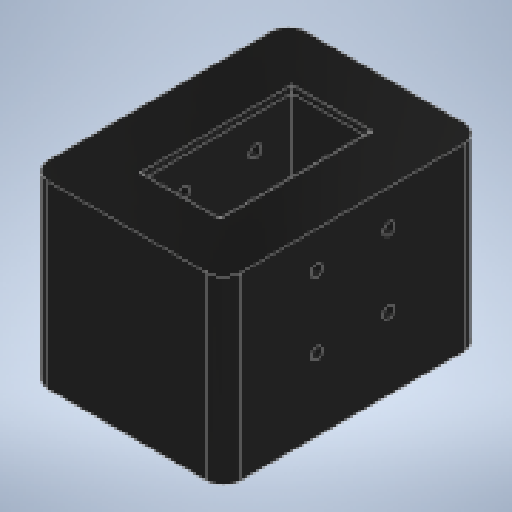
# Autodesk Inventor part: framefixpart1
Saved by Autodesk Inventor 2024 (Build 280153000, 153)
## iProperties
Created: 2025-05-28
Part Number: framefixpart1
Material: 一般
Document SubType Name: Modeling
Designer: kshau
Density: 1 g/cm^3
Appearance: 滑らか - 黒
Mass: 159.689 g
Surface Area: 260.007 cm^2
Volume: 159.689 cm^3
Author: kshau
Autodesk Inventor part; units mm, degrees
ref_plane "YZ Plane" through (0, 0, 0) normal (1, 0, 0) x (0, 1, 0)
ref_plane "XZ Plane" through (0, 0, 0) normal (0, 1, 0) x (-1, 0, 0)
ref_plane "XY Plane" through (0, 0, 0) normal (0, 0, 1) x (1, 0, 0)
sketch "スケッチ1" plane through (0, 0, 0) normal (0, 1, 0) x (-1, 0, 0)
  line L0 (0, 0) -> (53.8, 0)
  line L1 (53.8, 0) -> (53.8, -71.8)
  line L2 (53.8, -71.8) -> (0, -71.8)
  line L3 (0, -71.8) -> (0, 0)
  dimension "d0" = 53.8
  dimension "d1" = 71.8
  constraints: 8 end point, 2 parallel, 1 horizontal, 1 perpendicular
  measures "d0" distance of L0.start L0.end
  measures "d1" distance of L2.end L0.start
extrude "押し出し1" add sketch "スケッチ1" along normal blind 10
sketch "スケッチ2" plane through (0, 10, 0) normal (0, 1, 0) x (1, 0, 0)
  line L0 (-53.8, 71.8) -> (-53.8, 0) projected
  line L1 (-53.8, 0) -> (0, 0) projected
  line L2 (-26.9, 0) -> (-26.9, 71.8)
  line L3 (0, 71.8) -> (-53.8, 71.8) projected
  line L4 (-53.8, 35.9) -> (0, 35.9)
  line L5 (0, 0) -> (0, 71.8) projected
  line L6 (-26.9, 35.9) -> (-37.05, 35.9)
  line L7 (-37.05, 35.9) -> (-37.05, 56.05)
  line L8 (-37.05, 56.05) -> (-26.9, 56.05)
  line L9 (-26.9, 56.05) -> (-26.9, 35.9)
  line L10 (-37.05, 35.9) -> (-37.05, 15.75)
  line L11 (-37.05, 15.75) -> (-26.9, 15.75)
  line L12 (-16.75, 35.9) -> (-16.75, 56.05)
  line L13 (-16.75, 56.05) -> (-26.9, 56.05)
  line L14 (-16.75, 35.9) -> (-16.75, 15.75)
  line L15 (-16.75, 15.75) -> (-26.9, 15.75)
  dimension "d7" = 20.15
  dimension "d8" = 10.15
  constraints: 24 end point, 5 midpoint, 5 symmetric about line, 2 parallel, 1 horizontal, 1 perpendicular
  measures "d7" distance of L6.end L7.end
  measures "d8" distance of L7.end L8.end
extrude "押し出し2" add sketch "スケッチ2" along normal blind 40 contours L3 L2 L8 L7 L4 L0 | L4 L10 L11 L2 L1 L0 | L3 L5 L4 L12 L13 L2 | L2 L15 L14 L4 L5 L1
fillet "フィレット1" radius 5 4 edges at (0, 25, 0) (0, 25, -71.8) (-53.8, 25, -71.8) (-53.8, 25, 0)
sketch "スケッチ3" plane through (0, 0, -5) normal (1, 0, 0) x (0, 0, -1)
  line L0 (51.05, 50) -> (10.75, 50) projected
  line L1 (30.9, 50) -> (30.9, 0)
  line L2 (0, 0) -> (61.8, 0) projected
  line L3 (20.9, 50) -> (20.9, 0)
  line L4 (0, 50) -> (0, 0) projected
  line L5 (0, 10) -> (62, 10)
  line L6 (10.75, 10) -> (51.05, 10) projected
  point P0 (-5, 0)
  point P1 (20.9, 20)
  point P2 (20.9, 40)
  point P3 (40.9, 20)
  point P4 (40.9, 40)
  dimension "d12" = 10
  dimension "d13" = 10
  dimension "d14" = 10
  dimension "d15" = 20
  constraints: 6 end point, 3 point on line, 2 midpoint, 2 symmetric about line, 1 collinear, 1 vertical
  measures "d12" distance between parallel lines of L1 L3
  measures "d13" distance between parallel lines of L2 L5
  measures "d14" distance from line of L5 point (20.9, 20)
  measures "d15" distance of point (20.9, 20) point (20.9, 40)
hole "穴1" at (0, 20, -25.9) at (0, 40, -25.9) at (0, 40, -45.9) at (0, 20, -45.9) direction (-1, 0, 0) diameter 3.3 end through all
sketch "スケッチ4" plane through (0, 0, 0) normal (0, -1, 0) x (1, 0, 0)
  line L0 (-5, -71.8) -> (-48.8, -71.8) projected
  line L1 (-26.9, -71.8) -> (-26.9, 0)
  line L2 (-48.8, 0) -> (-5, 0) projected
  line L3 (-53.8, -66.8) -> (-53.8, -5) projected
  line L4 (-53.8, -35.9) -> (0, -35.9)
  line L5 (0, -5) -> (0, -66.8) projected
  point P0 (0, 0)
  point P1 (-26.9, -45.9)
  point P2 (-26.9, -25.9)
  dimension "d23" = 10
  dimension "d24" = 10
  constraints: 4 end point, 4 midpoint, 2 point on line
  measures "d23" distance from line of L4 point (-26.9, -25.9)
  measures "d24" distance from line of L4 point (-26.9, -45.9)
hole "穴2" at (-26.9, 0, -45.9) at (-26.9, 0, -25.9) direction (0, 1, 0) diameter 4.1 end through all
fillet "フィレット2" radius 1 4 edges at (-37.05, 50, -35.9) (-26.9, 50, -15.75) (-16.75, 50, -35.9) (-26.9, 50, -56.05)
sketch "スケッチ5" plane through (0, 0, 0) normal (0, -1, 0) x (1, 0, 0)
  circle A0 centre (-26.9, -25.9) radius 2.05 projected
  circle A1 centre (-26.9, -45.9) radius 2.05 projected
  line L0 (-26.9, -25.9) -> (-26.9, -45.9)
  line L1 (-26.9, -35.9) -> (-17.9, -35.9)
  line L2 (-17.9, -35.9) -> (-17.9, -42.9)
  line L3 (-17.9, -42.9) -> (-26.9, -42.9)
  line L4 (-26.9, -42.9) -> (-26.9, -35.9)
  line L5 (-17.9, -35.9) -> (-17.9, -28.9)
  line L6 (-17.9, -28.9) -> (-26.9, -28.9)
  line L7 (-35.9, -35.9) -> (-35.9, -42.9)
  line L8 (-35.9, -42.9) -> (-26.9, -42.9)
  line L9 (-35.9, -35.9) -> (-35.9, -28.9)
  line L10 (-35.9, -28.9) -> (-26.9, -28.9)
  point P0 (0, 0)
  dimension "d33" = 7
  dimension "d34" = 9
  constraints: 22 end point, 5 symmetric about line, 2 parallel, 1 horizontal, 1 midpoint, 1 perpendicular, 1 vertical
  measures "d33" distance of L1.end L2.end
  measures "d34" distance of L2.end L3.end
extrude "押し出し3" cut sketch "スケッチ5" against normal blind 10 contours L6 L5 L1 L0 | L0 L8 L7 L9 L10 | L1 L2 L3 L0
